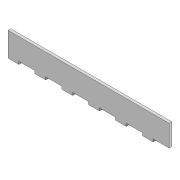
# Autodesk Inventor part: Divisória-22cm
Saved by Autodesk Inventor 2020 (Build 240168000, 168)
## iProperties
Created: 2021-09-21
Part Number: Divisória-22cm
Material: Generic
Document SubType Name: Modeling
Designer: pablo
Density: 1 g/cm^3
Appearance: Default
Author: pablo
Autodesk Inventor part; units mm, degrees
ref_plane "YZ Plane" through (0, 0, 0) normal (1, 0, 0) x (0, 1, 0)
ref_plane "XZ Plane" through (0, 0, 0) normal (0, 1, 0) x (-1, 0, 0)
ref_plane "XY Plane" through (0, 0, 0) normal (0, 0, 1) x (1, 0, 0)
sketch "Sketch1" plane through (0, 0, 0) normal (0, 0, 1) x (1, 0, 0)
  line L0 (-150, 20) -> (150, 20)
  line L1 (150, 20) -> (150, -20)
  line L2 (150, -20) -> (-150, -20)
  line L3 (-150, -20) -> (-150, 20)
  line L4 (-150, 20) -> (150, -20) construction
  line L5 (150, 20) -> (-150, -20) construction
  point P0 (0, 0)
  dimension "d0" = 300
  dimension "d1" = 40
  constraints: 12 end point, 2 midpoint, 2 parallel, 1 horizontal, 1 perpendicular
  measures "d0" distance of L1.end L2.end
  measures "d1" distance of L0.end L1.end
extrude "Base" add sketch "Sketch1" along normal blind 5
sketch "Sketch2" plane through (0, 0, 5) normal (0, 0, 1) x (1, 0, 0)
  line L0 (-150, -20) -> (150, -20) projected
  line L1 (-150, -20) -> (-130, -20)
  line L2 (-130, -20) -> (-130, -25)
  line L3 (-130, -25) -> (-150, -25)
  line L4 (-150, -25) -> (-150, -20)
  line L5 (-100, -20) -> (-80, -20)
  line L6 (-80, -20) -> (-80, -25)
  line L7 (-80, -25) -> (-100, -25)
  line L8 (-100, -25) -> (-100, -20)
  line L9 (-50, -20) -> (-30, -20)
  line L10 (-30, -20) -> (-30, -25)
  line L11 (-30, -25) -> (-50, -25)
  line L12 (-50, -25) -> (-50, -20)
  line L13 (0, -20) -> (20, -20)
  line L14 (20, -20) -> (20, -25)
  line L15 (20, -25) -> (0, -25)
  line L16 (0, -25) -> (0, -20)
  line L17 (50, -20) -> (70, -20)
  line L18 (70, -20) -> (70, -25)
  line L19 (70, -25) -> (50, -25)
  line L20 (50, -25) -> (50, -20)
  line L21 (100, -20) -> (120, -20)
  line L22 (120, -20) -> (120, -25)
  line L23 (120, -25) -> (100, -25)
  line L24 (100, -25) -> (100, -20)
  point P0 (0, 0)
  point P1 (20, -20)
  point P2 (-30, -20)
  point P3 (70, -20)
  point P4 (50, -20)
  point P5 (-100, -20)
  dimension "d4" = 20
  dimension "d5" = 5
  dimension "d8" = 50
  constraints: 48 end point, 2 horizontal, 2 parallel, 1 perpendicular, 40 other
  measures "d4" distance of L2.end L3.end
  measures "d5" distance of L1.end L2.end
  measures "d8" distance of L2.end L6.end
extrude "Encaixe" add sketch "Sketch2" against normal blind 5
body "Solid1"
